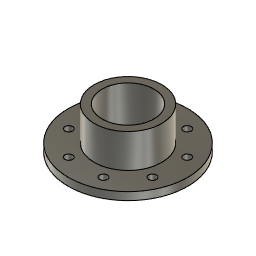
Part 16 (Autodesk Fusion 360 design; units mm, degrees)
Autodesk Fusion 360 part; units mm, degrees
note: some values were not read from the file. Chosen so that the rebuilt part matches the saved one: a direction. Set by a fixed rule: which sketch regions a step uses.
sketch "Sketch1" plane through (0, 0, 0) normal (0, 0, 1) x (1, 0, 0)
  circle A0 centre (0, 0) radius 115
  circle A1 centre (0, 0) radius 87.5 construction
  circle A2 centre (0, 0) radius 65
  circle A3 centre (0, 0) radius 50
  dimension "d1" = 230
  dimension "d2" = 175
  dimension "d3" = 130
  dimension "d4" = 100
  constraint coincident A0.centre A1.centre
  constraint concentric A0 A1
  constraint concentric A0 A2
  constraint concentric A1 A3
  measures "d1" diameter of A0
  measures "d2" diameter of A1
  measures "d3" diameter of A2
  measures "d4" diameter of A3
extrude "Extrude1" add sketch "Sketch1" along normal blind 15 contours A0
extrude "Extrude2" add sketch "Sketch1" along normal blind 80 contours A2
sketch "Sketch2" plane through (0, 0, 15) normal (0, 0, 1) x (-1, 0, 0)
  circle A0 centre (0, 0) radius 65
  circle A1 centre (0, 0) radius 115
  circle A2 centre (0, 0) radius 87.5
  line L0 (0, 0) -> (0, -122.0079) construction
  line L1 (0, 0) -> (50.2765, -121.3782) construction
  circle A3 centre (33.4848, -80.8395) radius 7.5
  dimension "d11" = 22.5
  dimension "d12" = 15
  constraint coincident A0.centre A1.centre
  constraint vertical L0
  constraint coincident A2 A3.centre
  constraint coincident L1 A3.centre
  measures "d11" angle of L0 L1
  measures "d12" diameter of A3
extrude "Extrude3" cut sketch "Sketch2" against normal through all contours A2 A3 | A2 A3 picked at (32.6894, -78.4443) picked at (34.4384, -83.1246)
pattern_circular "C-Pattern1" count 8 over 360 about axis through (0, 0, 0) along (0, 0, 1) of "Extrude3"
